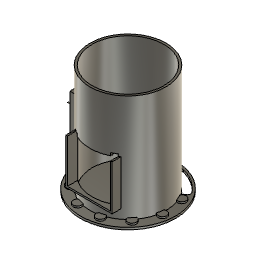
CoozieInnerShell v17 (Autodesk Fusion 360 design; units mm, degrees)
part number: Configuration 1
Autodesk Fusion 360 part; units mm, degrees
note: some values were not read from the file. Chosen so that the rebuilt part matches the saved one: where a step ends.
sketch "Sketch1" plane through (0, 0, 0) normal (0, 0, 1) x (1, 0, 0)
  circle A0 centre (0, 0) radius 33.5
  circle A1 centre (0, 0) radius 35.5
  dimension "d1" = 67
  dimension "shell_thickness" = 2
  constraint coincident A0.centre A1.centre
  measures "d1" diameter of A0
  measures "shell_thickness" distance of A0 A1
extrude "Extrude1" add sketch "Sketch1" along normal blind 100
sketch "Sketch2" plane through (0, 0, 0) normal (0, 0, 1) x (1, 0, 0)
  circle A0 centre (0, 0) radius 35.5
  circle A1 centre (0, 0) radius 44.5
  dimension "innerShellGap" = 9
  constraint coincident A0.centre A1.centre
  measures "innerShellGap" distance of A0 A1
extrude "Extrude3" add sketch "Sketch2" against normal blind 2 contours A0 | A1
sketch "Sketch4" plane through (0, 0, 0) normal (0, 0, 1) x (1, 0, 0)
  circle A0 centre (0, 38) radius 2.55
  circle A1 centre (0, 0) radius 44.5
  circle A2 centre (0, 38) radius 4.05
  dimension "d16" = 5.1
  dimension "d17" = 38
  dimension "d20" = 1.5
  constraint vertical A0.centre A1.centre
  constraint concentric A0 A2
  measures "d16" diameter of A0
  measures "d17" distance of A0.centre A1.centre
  measures "d20" distance of A0 A2
extrude "Extrude5" cut sketch "Sketch4" against normal blind 9 contours A0
extrude "Extrude6" add sketch "Sketch4" along normal blind 1.5 contours A0 | A2
pattern_circular "C-Pattern2" count 11 over 360 about axis through (0, 0, 0) along (0, 0, 1) of "Extrude5", "Extrude6"
ref_plane "WorkPlane1" through (0, -33.5, 27.8455) normal (0, 1, 0) x (1, 0, 0)
sketch "Sketch5" plane through (0, -33.5, 0) normal (0, 1, 0) x (1, 0, 0)
  line L0 (20.125, -50.25) -> (-20.125, -50.25)
  line L1 (-20.125, -50.25) -> (-20.125, -10)
  line L2 (-20.125, -10) -> (20.125, -10)
  line L3 (20.125, -10) -> (20.125, -50.25)
  line L4 (20.125, -50.25) -> (-20.125, -10) construction
  line L5 (-20.125, -50.25) -> (20.125, -10) construction
  line L6 (-44.5, 0) -> (44.5, 0)
  point P0 (0, -30.125)
  dimension "d26" = 40.25
  dimension "d27" = 40.25
  dimension "d28" = 10
  constraint horizontal L0
  constraint perpendicular L0 L1
  constraint parallel L0 L2
  constraint parallel L1 L3
  constraint coincident L4 P0
  constraint coincident L5 P0
  constraint vertical origin P0
  measures "d26" distance of L0.start L0.end
  measures "d27" distance of L0.end L1.end
  measures "d28" distance of L2 L6
extrude "Extrude7" cut sketch "Sketch5" along normal blind -55 and the other way blind -10
sketch "Sketch6" plane through (0, -33.5, 0) normal (0, 1, 0) x (1, 0, 0)
  line L0 (-20.125, -50.25) -> (-20.125, -10)
  line L1 (-20.125, -10) -> (20.125, -10)
  line L2 (20.125, -10) -> (20.125, -50.25)
  line L3 (20.125, -50.25) -> (-20.125, -50.25)
  line L4 (33.5, -100) -> (-33.5, -100)
  line L5 (33.5, 0) -> (-33.5, 0)
  line L6 (-20.125, -10) -> (-21.625, -10)
  line L7 (-21.625, -10) -> (-21.625, -50.659)
  line L8 (-21.625, -50.659) -> (-20.125, -50.659)
  line L9 (-20.125, -50.659) -> (-20.125, -10)
  line L10 (20.125, -10) -> (21.625, -10)
  line L11 (21.625, -10) -> (21.625, -50.659)
  line L12 (21.625, -50.659) -> (20.125, -50.659)
  line L13 (20.125, -50.659) -> (20.125, -10)
  line L14 (-21.625, -10) -> (21.625, -10)
  line L15 (21.625, -10) -> (21.625, -8.5)
  line L16 (21.625, -8.5) -> (-21.625, -8.5)
  line L17 (-21.625, -8.5) -> (-21.625, -10)
  dimension "d33" = 1.5
  dimension "d34" = 1.5
  dimension "d37" = 1.5
  constraint horizontal L6
  constraint vertical L7
  constraint horizontal L8
  constraint vertical L9
  constraint coincident L0.end L1.start
  constraint horizontal L10
  constraint vertical L11
  constraint horizontal L12
  constraint vertical L13
  constraint coincident L1.end L2.start
  constraint perpendicular L14 L15
  constraint parallel L14 L16
  constraint parallel L15 L17
  measures "d33" distance of L11.end L12.end
  measures "d34" distance of L7.end L8.end
  measures "d37" distance of L6.end L16.end
extrude "Extrude8" add sketch "Sketch6" along normal blind -3 and the other way blind -7.286 contours L0 L6 L7 L8 L9 L14 | L1 L6 L10 L14 L15 L16 L17 | L2 L10 L11 L12 L13 L14
extrude "Extrude16" cut sketch "Sketch1" along normal through all contours A0
ref_plane "WorkPlane2" through (0, 33.5, 30.4799) normal (0, -1, 0) x (-1, 0, 0)
sketch "Sketch10" plane through (0, 33.5, 0) normal (0, -1, 0) x (-1, 0, 0)
  circle A0 centre (0, -25) radius 4.1
  line L0 (-44.5, 0) -> (44.5, 0)
  circle A1 centre (0, -25) radius 5.6
  dimension "d48" = 8.2
  dimension "d49" = 25
  dimension "d50" = 1.5
  constraint vertical origin A0.centre
  constraint concentric A0 A1
  measures "d48" diameter of A0
  measures "d49" distance of A0.centre L0
  measures "d50" distance of A0 A1
extrude "Extrude10" cut sketch "Sketch10" along normal blind 10 and the other way blind 19 contours A0
extrude "Extrude11" add sketch "Sketch10" against normal blind 4
sketch "Sketch11" plane through (0, 37.5, 0) normal (0, 1, 0) x (-1, 0, 0)
  circle A0 centre (0, 25) radius 4.1
  circle A1 centre (0, 25) radius 5.6
  line L0 (-6, 18.5) -> (6, 18.5)
  line L1 (6, 18.5) -> (6, 34)
  line L2 (6, 34) -> (-6, 34)
  line L3 (-6, 34) -> (-6, 18.5)
  circle A2 centre (0, 25) radius 5.6
  point P0 (0, 34)
  point P1 (0, 25)
  dimension "d57" = 12
  dimension "d62" = 6.5
  dimension "d63" = 9
  constraint horizontal L0
  constraint vertical L1
  constraint horizontal L2
  constraint vertical L3
  constraint midpoint L2 P0
  constraint vertical P0 P1
  measures "d57" distance of L1.end L2.end
  measures "d62" distance of L0 P1
  measures "d63" distance of L2 P1
extrude "Extrude12" add sketch "Sketch11" along normal up to surface contours L0 L1 L2 L3 end surface at (-10.3013, 33.9725, 41.8795)
chamfer "Chamfer1" distance 1 angle 45 1 edges at (3.8225, 37.5, 26.4826)
sketch "Sketch12" plane through (0, -33.5, 0) normal (0, 1, 0) x (1, 0, 0)
  line L0 (20.125, -50.25) -> (-20.125, -50.25)
  line L1 (-20.125, -50.25) -> (-15.625, -50.25)
  line L2 (-15.625, -50.25) -> (-15.625, -52.75)
  line L3 (-15.625, -52.75) -> (-20.125, -52.75)
  line L4 (-20.125, -52.75) -> (-20.125, -50.25)
  line L5 (20.125, -50.25) -> (15.625, -50.25)
  line L6 (15.625, -50.25) -> (15.625, -52.75)
  line L7 (15.625, -52.75) -> (20.125, -52.75)
  line L8 (20.125, -52.75) -> (20.125, -50.25)
  dimension "d64" = 4.5
  dimension "d65" = 4.5
  dimension "d66" = 2.5
  dimension "d67" = 2.5
  constraint horizontal L1
  constraint vertical L2
  constraint horizontal L3
  constraint vertical L4
  constraint coincident L0.end L1.start
  constraint horizontal L5
  constraint vertical L6
  constraint horizontal L7
  constraint vertical L8
  constraint coincident L0.start L5.start
  measures "d64" distance of L2.end L3.end
  measures "d65" distance of L6.end L7.end
  measures "d66" distance of L0.end L3.end
  measures "d67" distance of L0.start L7.end
extrude "Extrude13" cut sketch "Sketch12" along normal blind -4 and the other way blind -6
ref_plane "WorkPlane3" through (-35.5, 0, 55.4852) normal (-1, 0, 0) x (0, 1, 0)
sketch "Sketch13" plane through (-35.5, 0, 0) normal (-1, 0, 0) x (0, -1, 0)
  line L0 (-17.78, 10) -> (17.78, 10)
  line L1 (17.78, 10) -> (17.78, 87.47)
  line L2 (17.78, 87.47) -> (-17.78, 87.47)
  line L3 (-17.78, 87.47) -> (-17.78, 10)
  line L4 (-17.78, 10) -> (17.78, 87.47) construction
  line L5 (17.78, 10) -> (-17.78, 87.47) construction
  line L6 (44.5, 0) -> (-44.5, 0)
  circle A0 centre (-16.51, 11.27) radius 0.5
  line L7 (17.78, 10) -> (-4.22, 10) construction
  line L8 (-4.22, 10) -> (-4.22, 17.5)
  line L9 (-4.22, 17.5) -> (17.78, 17.5)
  line L10 (17.78, 17.5) -> (17.78, 10) construction
  circle A1 centre (16.51, 18.87) radius 0.5
  circle A2 centre (-16.51, 86.2) radius 0.5
  circle A3 centre (16.51, 58.24) radius 0.5
  line L11 (17.78, 87.47) -> (-14.78, 87.47)
  line L12 (-14.78, 87.47) -> (-14.78, 69.47)
  line L13 (-14.78, 69.47) -> (17.78, 69.47)
  line L14 (17.78, 69.47) -> (17.78, 87.47)
  point P0 (0, 48.735)
  dimension "d74" = 10
  dimension "d76" = 1
  dimension "d77" = 1.27
  dimension "d78" = 1.27
  dimension "d79" = 22
  dimension "d80" = 7.5
  dimension "d81" = 1
  dimension "d82" = 8.87
  dimension "d83" = 1.27
  dimension "d84" = 1
  dimension "d85" = 74.93
  dimension "d86" = 1.27
  dimension "d87" = 1
  dimension "d88" = 1.27
  dimension "d89" = 39.37
  dimension "d90" = 18
  dimension "d91" = 3
  dimension "d92" = 33.02
  dimension "d93" = 1.27
  constraint horizontal L0
  constraint perpendicular L0 L1
  constraint parallel L0 L2
  constraint parallel L1 L3
  constraint coincident L4 P0
  constraint coincident L5 P0
  constraint vertical origin P0
  constraint horizontal L7
  constraint vertical L8
  constraint horizontal L9
  constraint vertical L10
  constraint horizontal L11
  constraint vertical L12
  constraint horizontal L13
  constraint vertical L14
  measures "d74" distance of L0 L6
  measures "d76" diameter of A0
  measures "d77" distance of L0 A0.centre
  measures "d78" distance of L3 A0.centre
  measures "d79" distance of L0.end L7.end
  measures "d80" distance of L0.end L9.end
  measures "d81" diameter of A1
  measures "d82" distance of L7 A1.centre
  measures "d83" distance of L1 A1.centre
  measures "d84" diameter of A2
  measures "d85" vertical distance of A0.centre A2.centre
  measures "d86" distance of L3 A2.centre
  measures "d87" diameter of A3
  measures "d88" distance of L1 A3.centre
  measures "d89" distance of A1.centre A3.centre
  measures "d90" distance of L1.end L13.end
  measures "d91" distance of L3 L12
  measures "d92" horizontal distance of A0.centre A1.centre
  measures "d93" distance of L2 A2.centre
extrude "Extrude14" add sketch "Sketch13" along normal blind 1 and the other way up to near side of body 1 contours L0 L1 L2 L3 L8 L9 L12 L13 | A0 | A1 | A2 | A3
extrude "Extrude15" add sketch "Sketch13" along normal blind 4 contours A0 | A1 | A2 | A3
sketch "Sketch14" plane through (0, 0, 0) normal (0, 0, 1) x (-1, 0, 0)
  circle A0 centre (0, 0) radius 44.5
  arc A1 (-21.7089, -28.0887) -> (-16.5322, -31.4156) centre (-20.5444, -31.9676) ccw
  arc A2 (-30.8923, -17.4905) -> (-21.7089, -28.0887) centre (0, 0) ccw
  arc A3 (-33.4486, -11.893) -> (-30.8923, -17.4905) centre (-34.566, -15.7858) ccw
  arc A4 (-35.4443, 1.9877) -> (-33.4486, -11.893) centre (0, 0) ccw
  arc A5 (-34.5686, 8.0787) -> (-35.4443, 1.9877) centre (-37.6132, 5.408) ccw
  arc A6 (-28.743, 20.8348) -> (-34.5686, 8.0787) centre (0, 0) ccw
  arc A7 (-24.7133, 25.4854) -> (-28.743, 20.8348) centre (-28.7185, 24.8847) ccw
  arc A8 (-12.916, 33.067) -> (-24.7133, 25.4854) centre (0, 0) ccw
  arc A9 (-7.0117, 34.8007) -> (-12.916, 33.067) centre (-10.7058, 36.4607) ccw
  arc A10 (7.0117, 34.8007) -> (-7.0117, 34.8007) centre (0, 0) ccw
  arc A11 (12.916, 33.067) -> (7.0117, 34.8007) centre (10.7058, 36.4607) ccw
  arc A12 (24.7133, 25.4854) -> (12.916, 33.067) centre (0, 0) ccw
  arc A13 (28.743, 20.8348) -> (24.7133, 25.4854) centre (28.7185, 24.8847) ccw construction
  arc A14 (34.5686, 8.0787) -> (28.743, 20.8348) centre (0, 0) ccw
  arc A15 (35.4443, 1.9877) -> (34.5686, 8.0787) centre (37.6132, 5.408) ccw
  arc A16 (33.4486, -11.893) -> (35.4443, 1.9877) centre (0, 0) ccw
  arc A17 (30.8923, -17.4905) -> (33.4486, -11.893) centre (34.566, -15.7858) ccw
  arc A18 (21.7089, -28.0887) -> (30.8923, -17.4905) centre (0, 0) ccw
  arc A19 (16.5322, -31.4156) -> (21.7089, -28.0887) centre (20.5444, -31.9676) ccw
  arc A20 (3.0768, -35.3664) -> (16.5322, -31.4156) centre (0, 0) ccw
  arc A21 (-3.0768, -35.3664) -> (3.0768, -35.3664) centre (0, -38) ccw
  arc A22 (-16.5322, -31.4156) -> (-3.0768, -35.3664) centre (0, 0) ccw
  arc A23 (28.743, 20.8348) -> (24.7133, 25.4854) centre (28.7185, 24.8847) ccw
  arc A24 (12.916, 33.067) -> (7.0117, 34.8007) centre (10.7058, 36.4607) ccw
  line L0 (0, 0) -> (36.5452, 25.391)
  line L1 (0, 0) -> (7.915, 43.7904)
  line L2 (0, 0) -> (-7.5593, -41.8223)
  line L3 (0, 0) -> (-34.9027, -24.2498)
  arc A25 (-34.9027, -24.2498) -> (-7.5593, -41.8223) centre (0, 0) ccw
  circle A26 centre (0, 0) radius 35.5
  circle A27 centre (0, 0) radius 44.5
  dimension "d107" = 7
  dimension "d112" = 71
  constraint coincident A0.centre A2.centre
  constraint tangent A11 L1
  constraint tangent A23 L0
  constraint parallel L0 L3
  constraint parallel L1 L2
  constraint concentric A0 A26
  constraint coincident A0 L1.end
  constraint coincident A0 L0.end
  constraint coincident L0.end A27
  measures "d107" distance of A25 A26
  measures "d112" diameter of A26
extrude "Extrude18" cut sketch "Sketch14" along normal blind 5 and the other way blind 15 contours A1 A2 A22 L2 L3 A25 A26 | A1 A26
fillet "Fillet1" radius 3 2 edges at (7.5593, 41.8223, -1) (34.9027, 24.2498, -1)
